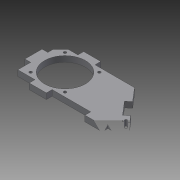
# Autodesk Inventor part: Controller_Side_A
Saved by Autodesk Inventor 2014 (Build 180170000, 170)
## iProperties
Created: 2014-11-10
Part Number: Controller_Side_A
Material: Generic
Document SubType Name: Modeling
Designer: ThatOtherGuy
Density: 1 g/cm^3
Appearance: Default
Author: ThatOtherGuy
Autodesk Inventor part; units mm, degrees
ref_plane "YZ Plane" through (0, 0, 0) normal (1, 0, 0) x (0, 1, 0)
ref_plane "XZ Plane" through (0, 0, 0) normal (0, 1, 0) x (-1, 0, 0)
ref_plane "XY Plane" through (0, 0, 0) normal (0, 0, 1) x (1, 0, 0)
sketch "Sketch1" plane through (0, 0, 0) normal (0, 0, 1) x (1, 0, 0)
  line L0 (0, 0) -> (125, 0)
  line L1 (125, 0) -> (125, 50)
  line L2 (125, 50) -> (0, 50)
  line L3 (0, 50) -> (0, 0)
  dimension "d0" = 125
  dimension "d1" = 50
  constraints: 8 end point, 2 parallel, 1 horizontal, 1 perpendicular
  measures "d0" distance between parallel lines of L3 L1
  measures "d1" distance of L2.end L0.start
extrude "Extrusion1" add sketch "Sketch1" along normal blind 6.731
sketch "Sketch4" plane through (0, 0, 0) normal (0, 0, -1) x (-1, 0, 0)
  line L0 (-125, 50) -> (0, 50) projected
  line L1 (-125, 0) -> (-125, 50) projected
  line L2 (-125, 4.3708) -> (-86.0388, 50)
  line L3 (-112.0129, 19.5805) -> (-106.8941, 15.2097)
  line L4 (-106.8941, 15.2097) -> (-93.907, 30.4195)
  line L5 (-93.907, 30.4195) -> (-99.0259, 34.7903)
  line L6 (0, 0) -> (-125, 0) projected
  line L7 (-125, 4.3708) -> (-119.8812, 0)
  circle A0 centre (-114.3237, 11.6915) radius 1.588
  dimension "d25" = 6.731
  dimension "d26" = 20
  dimension "d27" = 20
  dimension "d28" = 6.731
  dimension "d29" = 3.176
  dimension "d30" = 3.3655
  dimension "d31" = 7.5
  dimension "d40" = 60
  constraints: 10 end point, 5 point on line, 3 perpendicular, 1 centre point, 1 parallel
  measures "d25" distance of L4.end L5.end
  measures "d26" distance of L3.end L4.end
  measures "d27" distance of L2.start L3.start
  measures "d28" distance of L2.start L7.end
  measures "d29" diameter of A0
  measures "d30" distance from line of L2 A0.centre
  measures "d31" distance from line of L3 A0.centre
  measures "d40" distance of L2.start L2.end
extrude "LCD_Cut" cut sketch "Sketch4" against normal up to next contours L0 L2 L1 | L5 L4 L3 L2 | A0
sketch "Sketch2" plane through (0, 0, 6.731) normal (0, 0, 1) x (1, 0, 0)
  line L0 (0, 0) -> (125, 0) projected
  line L1 (125, 0) -> (125, 50) projected
  line L2 (0, 50) -> (0, 0) projected
  line L3 (20, 0) -> (40, 0)
  line L4 (40, 0) -> (40, -6.731)
  line L5 (40, -6.731) -> (20, -6.731)
  line L6 (20, -6.731) -> (20, 0)
  line L7 (105, 0) -> (85, 0)
  line L8 (85, 0) -> (85, -6.731)
  line L9 (85, -6.731) -> (105, -6.731)
  line L10 (105, -6.731) -> (105, 0)
  line L11 (0, 35) -> (-6.731, 35)
  line L12 (-6.731, 35) -> (-6.731, 15)
  line L13 (-6.731, 15) -> (0, 15)
  line L14 (0, 15) -> (0, 35)
  line L15 (86.0388, 50) -> (0, 50) projected
  line L16 (20, 50) -> (40, 50)
  line L17 (40, 50) -> (40, 56.731)
  line L18 (40, 56.731) -> (20, 56.731)
  line L19 (20, 56.731) -> (20, 50)
  point P0 (-6.731, 25)
  point P1 (0, 25)
  dimension "d4" = 6.731
  dimension "d5" = 20
  dimension "d6" = 20
  dimension "d7" = 20
  constraints: 32 end point, 8 parallel, 5 equal length, 4 horizontal, 4 perpendicular, 4 point on line, 2 collinear, 2 midpoint, 1 horizontal alignment
  measures "d4" distance of L3.end L4.end
  measures "d5" distance between parallel lines of L2 L6
  measures "d6" distance between parallel lines of L1 L10
  measures "d7" distance of L8.end L9.end
extrude "Tabs Pos" add sketch "Sketch2" against normal blind 6.731
sketch "Sketch3" plane through (0, 0, 0) normal (0, 0, -1) x (-1, 0, 0)
  line L0 (0, 50) -> (0, 0) projected
  line L1 (-86.0388, 50) -> (0, 50) projected
  line L2 (-20, -6.731) -> (-20, 0) projected
  circle A0 centre (-50, 45) radius 1.588
  circle A1 centre (-10, 45) radius 1.588
  circle A2 centre (-10, 5) radius 1.588
  circle A3 centre (-50, 5) radius 1.588
  line L3 (-50, 45) -> (-50, 5) construction
  line L4 (-10, 45) -> (-50, 45) construction
  line L5 (-50, 5) -> (-10, 45) construction
  circle A4 centre (-30, 25) radius 23.75
  point P0 (-150, 55)
  dimension "d10" = 3.176
  dimension "d11" = 40
  dimension "d12" = 5
  dimension "d13" = 50
  dimension "d14" = 10
  dimension "d15" = 47.5
  constraints: 6 end point, 5 centre point, 3 equal radius, 2 horizontal alignment, 2 perpendicular, 2 vertical alignment, 1 midpoint, 1 parallel, 1 other
  measures "d10" diameter of A0
  measures "d11" distance of L3.start L3.end
  measures "d13" distance of L0.start L0.end
  measures "d14" distance from line of L0 L4.start
  measures "d15" diameter of A4
extrude "Fan" cut sketch "Sketch3" against normal up to next
equation "\"d2\" = THICKB"
equation "\"d25\" = THICKB"
equation "\"d28\" = THICKB"
equation "\"d30\" = 0.5 * THICKB"
equation "\"d4\" = THICKB"
equation "\"d8\" = THICKB"
equation "\"d12\" = -0.5 * d11 + 0.5 * d13"
equation "\"THICKA\" = 3.175"
equation "\"THICKB\" = 6.731"
equation "\"THICKC\" = 12.7"
equation "\"THICKPLY\" = 5"
equation "\"MAGDIA\" = 9.5"
equation "\"BALLDIA\" = 12"
body "Solid1"
